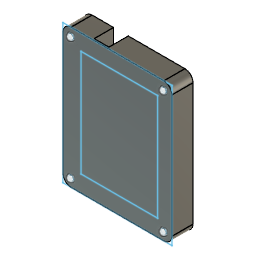
final (Autodesk Fusion 360 archive; units mm, degrees)
design "base_01_new"
part number: 2026-02-07-20-27-30-658
Autodesk Fusion 360 part; units mm, degrees
sketch "Sketch1" plane through (0, 0, 0) normal (0, 1, 0) x (1, 0, 0)
  line L0 (-90, -80) -> (-42.86, -80)
  line L1 (-42.86, -80) -> (-42.86, -14.63)
  line L2 (-42.86, -14.63) -> (-90, -14.63)
  line L3 (-90, -14.63) -> (-90, -80)
  line L4 (-34.1091, -89.705) -> (-101.2491, -89.705)
  line L5 (-101.2491, -89.705) -> (-101.2491, -4.335)
  line L6 (-101.2491, -4.335) -> (-34.1091, -4.335)
  line L7 (-34.1091, -4.335) -> (-34.1091, -89.705)
  circle A0 centre (-96.2491, -84.705) radius 1.45
  circle A1 centre (-39.1091, -84.705) radius 1.45
  circle A2 centre (-39.1091, -9.335) radius 1.45
  circle A3 centre (-96.2491, -9.335) radius 1.45
  dimension "d1" = 65.37
  dimension "d2" = 47.14
  dimension "d3" = 85.37
  dimension "d4" = 67.14
  dimension "d5" = 2.9
  dimension "d6" = 5
  dimension "d7" = 5
  dimension "d8" = 2.9
  dimension "d9" = 5
  dimension "d10" = 5
  dimension "d11" = 2.9
  dimension "d12" = 5
  dimension "d13" = 5
  dimension "d14" = 2.9
  dimension "d15" = 5
  dimension "d16" = 5
  constraint horizontal L0
  constraint vertical L1
  constraint horizontal L2
  constraint vertical L3
  constraint horizontal L4
  constraint vertical L5
  constraint horizontal L6
  constraint vertical L7
  measures "d1" distance of L0.start L2.end
  measures "d2" distance of L1 L3
  measures "d3" distance of L4.start L6.end
  measures "d4" distance of L5 L7
  measures "d5" diameter of A0
  measures "d6" distance of L5 A0.centre
  measures "d7" distance of L4 A0.centre
  measures "d8" diameter of A1
  measures "d9" distance of L7 A1.centre
  measures "d10" distance of L4 A1.centre
  measures "d11" diameter of A2
  measures "d12" distance of L6 A2.centre
  measures "d13" distance of L7 A2.centre
  measures "d14" diameter of A3
  measures "d15" distance of L5 A3.centre
  measures "d16" distance of L6 A3.centre
sketch "Sketch2" plane through (0, 0, 0) normal (0, 1, 0) x (1, 0, 0)
sketch "Sketch3" plane through (0, 0, 0) normal (0, 1, 0) x (1, 0, 0)
extrude "Extrude1" add sketch "Sketch1" along normal blind 13
extrude "Extrude2" add sketch "Sketch1" along normal blind 3 contours L0 L1 L2 L3
fillet "Fillet1" radius 5 1 edges at (-101.2491, 6.5, 89.705)
fillet "Fillet2" radius 5 1 edges at (-101.2491, 6.5, 4.335)
fillet "Fillet3" radius 5 1 edges at (-34.1091, 6.5, 4.335)
fillet "Fillet4" radius 5 1 edges at (-34.1091, 6.5, 89.705)
sketch "Sketch4" plane through (0, 13, 0) normal (0, 1, 0) x (-1, 0, 0)
  arc A0 (39.1091, 89.705) -> (34.1091, 84.705) centre (39.1091, 84.705) ccw
  line L0 (34.1091, 84.705) -> (34.1091, 9.335)
  arc A1 (34.1091, 9.335) -> (39.1091, 4.335) centre (39.1091, 9.335) ccw
  line L1 (39.1091, 4.335) -> (96.2491, 4.335)
  arc A2 (96.2491, 4.335) -> (101.2491, 9.335) centre (96.2491, 9.335) ccw
  line L2 (101.2491, 9.335) -> (101.2491, 84.705)
  arc A3 (101.2491, 84.705) -> (96.2491, 89.705) centre (96.2491, 84.705) ccw
  line L3 (96.2491, 89.705) -> (39.1091, 89.705)
  circle A4 centre (39.1091, 9.335) radius 1.45
  circle A5 centre (96.2491, 84.705) radius 1.45
  circle A6 centre (39.1091, 84.705) radius 1.45
  line L4 (90, 80) -> (90, 14.63)
  line L5 (90, 14.63) -> (42.86, 14.63)
  line L6 (42.86, 14.63) -> (42.86, 80)
  line L7 (42.86, 80) -> (90, 80)
  circle A7 centre (96.2491, 9.335) radius 1.45
  line L8 (74, 89.705) -> (83.03, 89.705)
  line L9 (83.03, 89.705) -> (83.03, 80)
  line L10 (83.03, 80) -> (74, 80)
  line L11 (74, 80) -> (74, 89.705)
  dimension "d29" = 9.03
  constraint horizontal L8
  constraint vertical L9
  constraint horizontal L10
  constraint vertical L11
  constraint coincident L7 L9.end
  constraint coincident L3 L8.start
  measures "d29" distance of L9 L11
extrude "Extrude3" cut sketch "Sketch4" against normal blind 12 contours L3 L7 L8 L9 L10 L11
